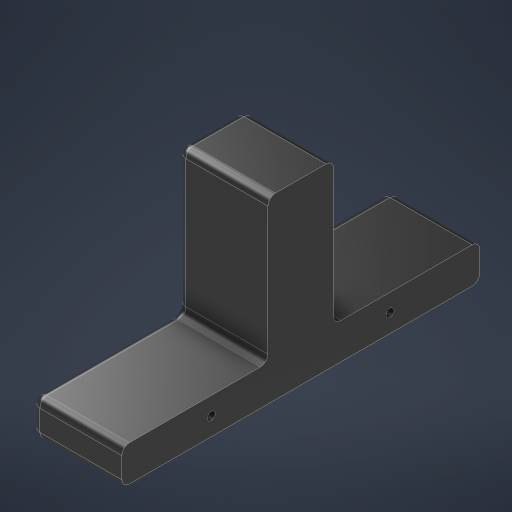
# Autodesk Inventor part: brain mount
Saved by Autodesk Inventor 2024 (Build 280153000, 153)
## iProperties
Created: 2023-12-20
Part Number: brain mount
Material: Generic
Document SubType Name: Modeling
Designer: elite
Density: 1 g/cm^3
Appearance: Glossy - Black
Author: elite
Autodesk Inventor part; units mm, degrees
ref_plane "YZ Plane" through (0, 0, 0) normal (1, 0, 0) x (0, 1, 0)
ref_plane "XZ Plane" through (0, 0, 0) normal (0, 1, 0) x (-1, 0, 0)
ref_plane "XY Plane" through (0, 0, 0) normal (0, 0, 1) x (1, 0, 0)
sketch "Sketch1" plane through (0, 0, 0) normal (1, 0, 0) x (0, 1, 0)
  line L0 (0, 0) -> (15.24, 0)
  line L1 (15.24, 0) -> (15.24, -152.4)
  line L2 (15.24, -152.4) -> (0, -152.4)
  line L3 (0, -152.4) -> (0, 0)
  line L4 (15.24, -76.2) -> (0, -76.2)
  line L5 (7.62, -76.2) -> (7.62, -114.3)
  line L6 (7.62, -76.2) -> (7.62, -38.1)
  circle A0 centre (7.62, -38.1) radius 1.778
  circle A1 centre (7.62, -114.3) radius 1.778
  line L7 (0, -76.2) -> (76.2, -76.2)
  line L8 (76.2, -76.2) -> (76.2, -90.17)
  line L9 (76.2, -90.17) -> (76.2, -62.23)
  line L10 (76.2, -62.23) -> (0, -62.23)
  line L11 (0, -62.23) -> (0, -90.17)
  line L12 (0, -90.17) -> (76.2, -90.17)
  line L13 (76.2, -90.17) -> (76.2, -62.23)
  point P0 (15.24, -62.23)
  point P1 (15.24, -90.17)
  dimension "d0" = 152.4
  dimension "d1" = 15.24
  dimension "d2" = 38.1
  dimension "d3" = 38.1
  dimension "d4" = 3.556
  dimension "d5" = 3.556
  dimension "d6" = 76.2
  dimension "d7" = 13.97
  dimension "d8" = 27.94
  constraints: 28 end point, 4 parallel, 3 midpoint, 3 perpendicular, 3 point on line, 2 centre point, 2 coincident, 2 horizontal, 2 vertical
  measures "d0" distance of L2.end L0.start
  measures "d1" distance of L0.start L0.end
  measures "d2" distance of L5.start L5.end
  measures "d3" distance of L5.start L6.end
  measures "d4" diameter of A0
  measures "d5" diameter of A1
  measures "d6" distance of L4.end L7.end
  measures "d7" distance of L7.end L8.end
  measures "d8" distance of L8.end L9.end
extrude "Extrusion1" add sketch "Sketch1" along normal blind 38.1
fillet "Fillet1" radius 3.175 17 edges at (0, 15.24, -31.115) (0, 7.62, 0) (0, 0, -76.2) (0, 7.62, -152.4) (0, 15.24, -121.285) (0, 45.72, -90.17) (0, 76.2, -69.215) (0, 76.2, -83.185) (0, 45.72, -62.23) (19.05, 15.24, 0) (19.05, 76.2, -62.23) (19.05, 15.24, -62.23) (19.05, 76.2, -90.17) (19.05, 15.24, -90.17) (19.05, 15.24, -152.4) (19.05, 0, -152.4) (19.05, 0, 0)
body "Solid1"
